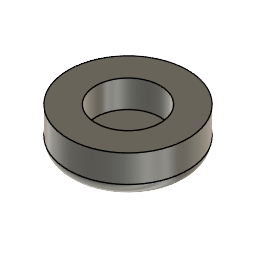
Cap 4 (Autodesk Fusion 360 design; units mm, degrees)
Autodesk Fusion 360 part; units mm, degrees
sketch "Sketch1" plane through (0, 0, 0) normal (0, 0, 1) x (1, 0, 0)
  circle A0 centre (0, 0) radius 3.55
  circle A1 centre (0, 0) radius 6.55
  dimension "d1" = 7.1
  dimension "d2" = 3
  constraint coincident A0.centre A1.centre
  measures "d1" diameter of A0
extrude "Extrude1" add sketch "Sketch1" along normal blind 3
extrude "Extrude3" add sketch "Sketch1" against normal blind 1.5 contours A0 | A1
fillet "Fillet1" radius 1.5 1 edges at (-6.1067, 2.3686, -1.5)
